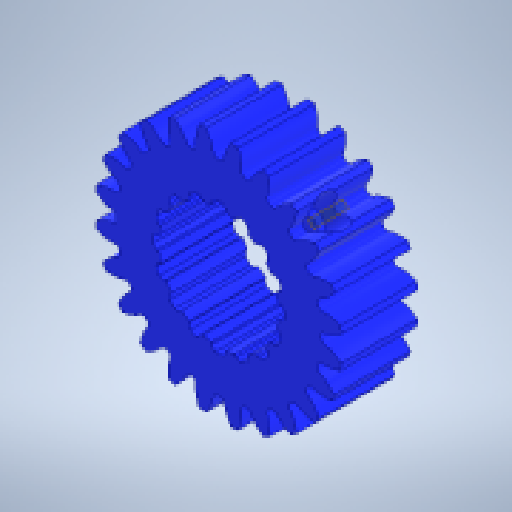
# Autodesk Inventor part: шестреня_12.12
Saved by Autodesk Inventor 2023.1 (Build 271208000, 208)
## iProperties
Created: 2025-12-12
Part Number: шестреня_12.12
Material: Generic
Document SubType Name: Modeling
Designer: DELL
Density: 1 g/cm^3
Appearance: Синий — малярная краска — глянцевая
Author: DELL
Autodesk Inventor part; units mm, degrees
ref_plane "YZ Plane" through (0, 0, 0) normal (1, 0, 0) x (0, 1, 0)
ref_plane "XZ Plane" through (0, 0, 0) normal (0, 1, 0) x (-1, 0, 0)
ref_plane "XY Plane" through (0, 0, 0) normal (0, 0, 1) x (1, 0, 0)
sketch "Sketch1" plane through (0, 0, 0) normal (0, 0, 1) x (1, 0, 0)
  spline S0 degree 3 poles (-2.683, 25.8612) (-2.6177, 25.7693) (-2.4871, 25.5856) (-2.3012, 25.3031) (-2.1229, 25.0157) (-1.9537, 24.7229) (-1.7941, 24.4247) (-1.6452, 24.1211) (-1.5081, 23.8119) (-1.3843, 23.4971) (-1.2774, 23.1763) (-1.1862, 22.8501) (-1.1454, 22.571) (-1.0953, 22.351) (-1.0419, 22.1903) (-0.9722, 22.0362) (-0.8862, 21.89) (-0.7938, 21.783) (-0.7126, 21.7048) (-0.6444, 21.6545) (-0.5738, 21.6077) (-0.4972, 21.5717) (-0.4191, 21.539) (-0.3368, 21.5189) (-0.2537, 21.5027) (-0.1408, 21.4983) (0, 21.5011) (0.1408, 21.4983) (0.2537, 21.5027) (0.3368, 21.5189) (0.4191, 21.539) (0.4972, 21.5717) (0.5738, 21.6077) (0.6444, 21.6545) (0.7126, 21.7048) (0.7938, 21.783) (0.8862, 21.89) (0.9722, 22.0362) (1.0419, 22.1903) (1.0953, 22.351) (1.1454, 22.571) (1.1862, 22.8501) (1.2774, 23.1763) (1.3843, 23.4971) (1.5081, 23.8119) (1.6452, 24.1211) (1.7941, 24.4247) (1.9537, 24.7229) (2.1229, 25.0157) (2.3012, 25.3031) (2.4871, 25.5856) (2.6177, 25.7693) (2.683, 25.8612) knots 0 0 0 0 0.033813 0.067626 0.101438 0.135251 0.169064 0.202876 0.236688 0.270499 0.304309 0.338116 0.371923 0.388829 0.405731 0.422625 0.439519 0.456403 0.464858 0.473311 0.481763 0.490215 0.498666 0.507118 0.51557 0.524022 0.540929 0.557835 0.566287 0.574739 0.583191 0.591642 0.600094 0.608546 0.616999 0.625454 0.642338 0.659232 0.676126 0.693028 0.709934 0.743742 0.777548 0.811358 0.845169 0.878981 0.912793 0.946606 0.980419 1.014232 1.048044 1.081857 1.081857 1.081857 1.081857
  circle A0 centre (0, 0) radius 21.5 construction
  circle A1 centre (0, 0) radius 22.5526 construction
  circle A2 centre (0, 0) radius 24 construction
  circle A3 centre (0, 0) radius 26
  point P0 (-2.4888, 25.5844)
  point P1 (-2.3025, 25.3022)
  point P2 (-2.1244, 25.0148)
  point P3 (-1.9553, 24.722)
  point P4 (-1.7959, 24.4238)
  point P5 (-1.6472, 24.1202)
  point P6 (-1.5103, 23.811)
  point P7 (-1.3871, 23.4961)
  point P8 (-1.28, 23.1754)
  point P9 (-1.1932, 22.8487)
  point P10 (-1.1314, 22.5163)
  point P11 (-1.0927, 22.3517)
  point P12 (-1.0392, 22.1914)
  point P13 (-0.9695, 22.0375)
  point P14 (-0.8821, 21.8929)
  point P15 (-0.7729, 21.7641)
  point P16 (-0.7114, 21.7062)
  point P17 (-0.644, 21.6551)
  point P18 (-0.5728, 21.6095)
  point P19 (-0.497, 21.5722)
  point P20 (-0.4184, 21.5411)
  point P21 (-0.3367, 21.5196)
  point P22 (-0.2534, 21.5049)
  point P23 (-0.1691, 21.5)
  point P24 (0, 21.5)
  point P25 (0.1691, 21.5)
  point P26 (0.2534, 21.5049)
  point P27 (0.3367, 21.5196)
  point P28 (0.4184, 21.5411)
  point P29 (0.497, 21.5722)
  point P30 (0.5728, 21.6095)
  point P31 (0.644, 21.6551)
  point P32 (0.7114, 21.7062)
  point P33 (0.7729, 21.7641)
  point P34 (0.8821, 21.8929)
  point P35 (0.9695, 22.0375)
  point P36 (1.0392, 22.1914)
  point P37 (1.0927, 22.3517)
  point P38 (1.1314, 22.5163)
  point P39 (1.1932, 22.8487)
  point P40 (1.28, 23.1754)
  point P41 (1.3871, 23.4961)
  point P42 (1.5103, 23.811)
  point P43 (1.6472, 24.1202)
  point P44 (1.7959, 24.4238)
  point P45 (1.9553, 24.722)
  point P46 (2.1244, 25.0148)
  point P47 (2.3025, 25.3022)
  point P48 (2.4888, 25.5844)
  constraints: 4 centre point, 2 point on circle, 107 other
extrude "Выдавливание1" add sketch "Sketch1" against normal blind 16
sketch "Эскиз3" plane through (0, 0, 0) normal (0, 0, 1) x (1, 0, 0)
  circle A0 centre (0, 0) radius 12.65
  dimension "d12" = 25.3
  constraints: 1 centre point, 1 coincident
  measures "d12" diameter of A0
extrude "Выдавливание4" cut sketch "Эскиз3" against normal blind 16.2
extrude "Выдавливание2" cut sketch "Sketch1" against normal blind 16.2 contours A3 S0 picked at (-0.3163, 24.8409)
pattern_circular "Круговой массив1" count 24 over 360 about axis through (0, 0, 0) along (0, 0, -1) of "Выдавливание2"
sketch "Эскиз2" plane through (0, 0, 0) normal (0, 0, 1) x (1, 0, 0)
  line L0 (-11.4, -1.5) -> (-13.1, -1.5)
  line L1 (-13.9, -1.5) -> (-13.9, -0.75) construction
  line L2 (-13.9, 1.5) -> (-13.1, 1.5) construction
  line L3 (-11.4, 1.5) -> (-11.4, -1.5)
  circle A0 centre (0, 0) radius 12.65 projected
  line L4 (-11.4, -1.5) -> (-13.9, 1.5) construction
  line L5 (-13.9, -1.5) -> (-11.4, 1.5) construction
  line L6 (-13.9, 0) -> (-11.4, 0) construction
  line L7 (-13.9, 0) -> (-13.9, 0.75)
  line L8 (-13.9, -0.75) -> (-13.1, -1.5)
  line L9 (-13.1, -1.5) -> (-13.1, 1.5) construction
  line L10 (-13.9, 0.75) -> (-13.1, 1.5)
  line L11 (-13.1, 1.5) -> (-11.4, 1.5)
  line L12 (-13.1, -1.5) -> (-13.9, -1.5) construction
  line L13 (-13.9, 0.75) -> (-13.9, 1.5) construction
  line L14 (-13.9, -0.75) -> (-13.9, 0)
  point P0 (-12.65, 0)
  dimension "d21" = 2.5
  dimension "d22" = 3
  dimension "d23" = 0.8
  constraints: 30 end point, 10 perpendicular, 8 parallel, 3 midpoint, 2 horizontal, 1 horizontal alignment, 1 other
  measures "d21" distance of L2.start L3.start
  measures "d22" distance of L1.start L2.start
  measures "d23" distance of L1.start L0.end
extrude "Выдавливание3" cut sketch "Эскиз2" against normal blind 16.2 contours L0 A0 L11 L3 | L0 L8 L14 L7 L10 L11 A0 picked at (-11.8134, -0.167)
pattern_circular "Круговой массив2" count 16 over 360 about axis through (0, 0, 0) along (0, 0, -1) of "Выдавливание3"
sketch "Эскиз5" plane through (9.2985, 10.3591, 0) normal (-0.7071068, -0.7071068, 0) x (-0.7071068, 0.7071068, 0)
  line L0 (0, 0) -> (-1.5, 0) construction
  line L1 (0, 0) -> (0, 16) construction
  line L2 (-1.5, 16) -> (0, 16) construction
  line L3 (-1.5, 0) -> (-1.5, 16) construction
  circle A0 centre (-0.75, 6) radius 1.6
  line L4 (0.75, 0) -> (0, 0) projected
  point P0 (-0.75, 0)
  point P1 (0.375, 0)
  dimension "d24" = 3.2
  dimension "d34" = 6
  constraints: 2 end point, 1 centre point, 1 midpoint
  measures "d24" diameter of A0
  measures "d34" vertical distance of point (0.375, 0) A0.centre
extrude "Выдавливание5" cut sketch "Эскиз5" along normal blind 5 and the other way blind 10
ref_plane "РабПлоскость1" through (20.2586, 19.1979, 0) normal (-0.7071068, -0.7071068, 0) x (-0.7071068, 0.7071068, 0)
sketch "Эскиз6" plane through (20.2586, 19.1979, 0) normal (-0.7071068, -0.7071068, 0) x (-0.7071068, 0.7071068, 0)
  line L0 (2.2982, 5.5961) -> (2.2982, 6.4039) projected
  arc A0 (-0.7982, 6.4039) -> (-0.7982, 5.5961) centre (0.75, 6) ccw projected
  circle A1 centre (0.75, 6) radius 3.25
  point P0 (0.75, 0)
  dimension "d31" = 6.5
  constraints: 2 horizontal alignment, 1 centre point, 1 coincident
  measures "d31" diameter of A1
extrude "Выдавливание6" cut sketch "Эскиз6" along normal blind 10
equation "\"Модуль\" = 2"
equation "\"Угол_зацепления\" = 20deg"
equation "\"Зазор_профиля_зуба\" = 0.25"
equation "\"Радиус_закругления_зуба\" = 0.35"
equation "\"Диаметр_головки\" = 52"
equation "\"Диаметр_впадин\" = 43"
equation "\"Основной_диаметр\" = 45.10525"
equation "\"Средний_диаметр\" = 48"
equation "\"Ширина_грани\" = 16.2"
equation "\"Коэффициент_смещения\" = 0"
equation "\"Изменение_высоты_головки_зуба\" = 0"
equation "\"Окружной_шаг\" = 6.283185"
equation "\"Общий_сдвиг_инструмента\" = 0"
equation "\"Внутренний\" = 0"
